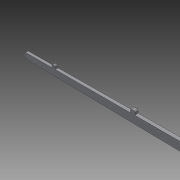
# Autodesk Inventor part: front_upper_brace
Saved by Autodesk Inventor 2014 (Build 180170000, 170)
## iProperties
Created: 2014-04-01
Part Number: front_upper_brace
Material: Plywood, Finish
Document SubType Name: Modeling
Designer: buben
Density: 0.552 g/cm^3
Appearance: Plywood - New
Author: buben
Autodesk Inventor part; units mm, degrees
ref_plane "YZ Plane" through (0, 0, 0) normal (1, 0, 0) x (0, 1, 0)
ref_plane "XZ Plane" through (0, 0, 0) normal (0, 1, 0) x (-1, 0, 0)
ref_plane "XY Plane" through (0, 0, 0) normal (0, 0, 1) x (1, 0, 0)
sketch "Sketch1" plane through (0, 0, 0) normal (0, 1, 0) x (-1, 0, 0)
  line L0 (0, 0) -> (-336, 0)
  line L1 (-336, 0) -> (-336, -15)
  line L2 (-336, -15) -> (0, -15)
  line L3 (0, -15) -> (0, 0)
  dimension "d0" = 15
  dimension "d1" = 336
  constraints: 8 end point, 2 parallel, 1 horizontal, 1 perpendicular
  measures "d0" distance of L2.end L0.start
  measures "d1" distance of L0.start L0.end
extrude "Extrusion1" add sketch "Sketch1" along normal blind 6.5
sketch "Sketch2" plane through (0, 6.5, 0) normal (0, 1, 0) x (1, 0, 0)
  line L0 (0, 0) -> (336, 0) projected
  line L1 (336, 0) -> (336, 15) projected
  line L2 (0, 15) -> (0, 0) projected
  line L3 (0, 12) -> (-4.5, 12)
  line L4 (-6.5, 10) -> (-6.5, 6)
  line L5 (-4.5, 4) -> (0, 4)
  line L6 (0, 4) -> (0, 12)
  line L7 (336, 12) -> (340.5, 12)
  line L8 (342.5, 10) -> (342.5, 6)
  line L9 (340.5, 4) -> (336, 4)
  line L10 (336, 4) -> (336, 12)
  line L11 (80, 0) -> (88, 0)
  line L12 (88, 0) -> (88, -4.5)
  line L13 (86, -6.5) -> (82, -6.5)
  line L14 (80, -4.5) -> (80, 0)
  line L15 (248, 0) -> (256, 0)
  line L16 (256, 0) -> (256, -4.5)
  line L17 (254, -6.5) -> (250, -6.5)
  line L18 (248, -4.5) -> (248, 0)
  arc A0 (-4.5, 12) -> (-6.5, 10) centre (-4.5, 10) ccw
  arc A1 (-6.5, 6) -> (-4.5, 4) centre (-4.5, 6) ccw
  arc A2 (80, -4.5) -> (82, -6.5) centre (82, -4.5) ccw
  arc A3 (86, -6.5) -> (88, -4.5) centre (86, -4.5) ccw
  arc A4 (248, -4.5) -> (250, -6.5) centre (250, -4.5) ccw
  arc A5 (254, -6.5) -> (256, -4.5) centre (254, -4.5) ccw
  arc A6 (340.5, 4) -> (342.5, 6) centre (340.5, 6) ccw
  arc A7 (342.5, 10) -> (340.5, 12) centre (340.5, 10) ccw
  dimension "d4" = 2
  dimension "d5" = 8
  dimension "d6" = 8
  dimension "d7" = 8
  dimension "d8" = 8
  dimension "d9" = 6.5
  dimension "d10" = 6.5
  dimension "d11" = 6.5
  dimension "d12" = 4
  dimension "d13" = 80
  dimension "d14" = 80
  constraints: 32 end point, 16 point on circle, 16 tangent, 8 centre point, 8 parallel, 7 equal radius, 4 horizontal, 4 perpendicular, 4 point on line, 2 collinear
  measures "d4" radius of A0
  measures "d5" distance between parallel lines of L5 L3
  measures "d6" distance between parallel lines of L12 L14
  measures "d7" distance between parallel lines of L16 L18
  measures "d8" distance between parallel lines of L9 L7
  measures "d9" distance between parallel lines of L4 L2
  measures "d10" distance between parallel lines of L0 L13
  measures "d11" distance between parallel lines of L1 L8
  measures "d12" distance between parallel lines of L0 L5
  measures "d13" distance between parallel lines of L2 L14
  measures "d14" distance between parallel lines of L1 L16
extrude "Extrusion2" add sketch "Sketch2" against normal blind 6.5
equation "\"d6\" = d5"
equation "\"d7\" = d6"
equation "\"d8\" = d7"
equation "\"d10\" = d9"
equation "\"d11\" = d9"
equation "\"d14\" = d13"
body "Solid1"
